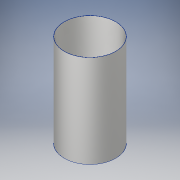
# Autodesk Inventor part: 55K mini shield
Saved by Autodesk Inventor 2018 (Build 220112000, 112)
## iProperties
Created: 2018-10-16
Part Number: 55K mini shield
Material: Aluminum 6061
Document SubType Name: Modeling
Designer: freyja
Density: 2.7 g/cm^3
Appearance: Aluminum - Flat
Author: freyja
Autodesk Inventor part; units mm, degrees
ref_plane "YZ Plane" through (0, 0, 0) normal (1, 0, 0) x (0, 1, 0)
ref_plane "XZ Plane" through (0, 0, 0) normal (0, 1, 0) x (-1, 0, 0)
ref_plane "XY Plane" through (0, 0, 0) normal (0, 0, 1) x (1, 0, 0)
sketch "Sketch1" plane through (0, 0, 0) normal (0, 1, 0) x (-1, 0, 0)
  circle A0 centre (0, 0) radius 133.35
  circle A1 centre (0, 0) radius 134.239
  dimension "d0" = 266.7
  dimension "d1" = 268.478
  constraints: 2 centre point, 2 coincident
  measures "d0" diameter of A0
  measures "d1" diameter of A1
extrude "Extrusion1" add sketch "Sketch1" along normal blind 482.6
body "Solid1"
